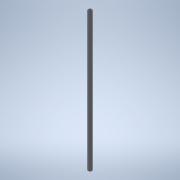
# Autodesk Inventor part: 20-4040_2m
Saved by Autodesk Inventor 2021 (Build 250183000, 183)
## iProperties
Created: 2014-04-23
Part Number: 20-4040_2m
Material: Generic
Document SubType Name: Modeling
Designer: Ross Bowman
Density: 1 g/cm^3
Engineer: Ross Bowman
Catalog Web Link: 8020.net
Vendor: 80/20 Inc.
Appearance: Default
Company: 80/20 Inc.
Material: 6105-T5 Aluminum
Author: Ross Bowman
Keywords: 80/20 , 8020 , T-Slot , Extrusion
Autodesk Inventor part; units mm, degrees
ref_plane "YZ Plane" through (0, 0, 0) normal (1, 0, 0) x (0, 1, 0)
ref_plane "XZ Plane" through (0, 0, 0) normal (0, 1, 0) x (-1, 0, 0)
ref_plane "XY Plane" through (0, 0, 0) normal (0, 0, 1) x (1, 0, 0)
sketch "Sketch1" plane through (0, 0, 0) normal (0, 0, 1) x (1, 0, 0)
  arc A0 (-12.1249, -12.3045) -> (-10.804, -11.9351) centre (-11.5684, -11.748) ccw
  line L0 (-12.3045, -12.1249) -> (-12.1249, -12.3045)
  arc A1 (-11.9351, -10.804) -> (-12.3045, -12.1249) centre (-11.748, -11.5684) ccw
  arc A2 (-11.9351, -9.196) -> (-11.9351, -10.804) centre (-10, -10) ccw
  arc A3 (-12.3045, -7.8751) -> (-11.9351, -9.196) centre (-11.748, -8.4316) ccw
  line L1 (-12.1249, -7.6955) -> (-12.3045, -7.8751)
  arc A4 (-10.804, -8.0649) -> (-12.1249, -7.6955) centre (-11.5684, -8.252) ccw
  arc A5 (-9.196, -8.0649) -> (-10.804, -8.0649) centre (-10, -10) ccw
  arc A6 (-7.8751, -7.6955) -> (-9.196, -8.0649) centre (-8.4316, -8.252) ccw
  line L2 (-7.6955, -7.8751) -> (-7.8751, -7.6955)
  arc A7 (-8.0649, -9.196) -> (-7.6955, -7.8751) centre (-8.252, -8.4316) ccw
  arc A8 (-8.0649, -10.804) -> (-8.0649, -9.196) centre (-10, -10) ccw
  arc A9 (-7.6955, -12.1249) -> (-8.0649, -10.804) centre (-8.252, -11.5684) ccw
  line L3 (-7.8751, -12.3045) -> (-7.6955, -12.1249)
  arc A10 (-9.196, -11.9351) -> (-7.8751, -12.3045) centre (-8.4316, -11.748) ccw
  arc A11 (-10.804, -11.9351) -> (-9.196, -11.9351) centre (-10, -10) ccw
  arc A12 (-2.505, -17.992) -> (-1.997, -18.5) centre (-1.997, -17.992) ccw
  line L4 (-2.505, -16.6448) -> (-2.505, -17.992)
  arc A13 (-2.505, -16.6448) -> (-2.6538, -16.2856) centre (-3.013, -16.6448) ccw
  line L5 (-6.1962, -12.7431) -> (-2.6538, -16.2856)
  arc A14 (-6.345, -12.3839) -> (-6.1962, -12.7431) centre (-5.837, -12.3839) ccw
  line L6 (-6.345, -7.488) -> (-6.345, -12.3839)
  arc A15 (-6.345, -7.488) -> (-7.488, -6.345) centre (-7.488, -7.488) ccw
  line L7 (-12.3839, -6.345) -> (-7.488, -6.345)
  arc A16 (-12.7431, -6.1962) -> (-12.3839, -6.345) centre (-12.3839, -5.837) ccw
  line L8 (-16.2856, -2.6538) -> (-12.7431, -6.1962)
  arc A17 (-16.2856, -2.6538) -> (-16.6448, -2.505) centre (-16.6448, -3.013) ccw
  line L9 (-17.992, -2.505) -> (-16.6448, -2.505)
  arc A18 (-18.5, -1.997) -> (-17.992, -2.505) centre (-17.992, -1.997) ccw
  line L10 (-18.5, 1.997) -> (-18.5, -1.997)
  arc A19 (-17.992, 2.505) -> (-18.5, 1.997) centre (-17.992, 1.997) ccw
  line L11 (-16.6448, 2.505) -> (-17.992, 2.505)
  arc A20 (-16.6448, 2.505) -> (-16.2856, 2.6538) centre (-16.6448, 3.013) ccw
  line L12 (-12.7431, 6.1962) -> (-16.2856, 2.6538)
  arc A21 (-12.3839, 6.345) -> (-12.7431, 6.1962) centre (-12.3839, 5.837) ccw
  line L13 (-7.488, 6.345) -> (-12.3839, 6.345)
  arc A22 (-7.488, 6.345) -> (-6.345, 7.488) centre (-7.488, 7.488) ccw
  line L14 (-6.345, 12.3839) -> (-6.345, 7.488)
  arc A23 (-6.1962, 12.7431) -> (-6.345, 12.3839) centre (-5.837, 12.3839) ccw
  line L15 (-2.6538, 16.2856) -> (-6.1962, 12.7431)
  arc A24 (-2.6538, 16.2856) -> (-2.505, 16.6448) centre (-3.013, 16.6448) ccw
  line L16 (-2.505, 17.992) -> (-2.505, 16.6448)
  arc A25 (-1.997, 18.5) -> (-2.505, 17.992) centre (-1.997, 17.992) ccw
  line L17 (1.997, 18.5) -> (-1.997, 18.5)
  arc A26 (2.505, 17.992) -> (1.997, 18.5) centre (1.997, 17.992) ccw
  line L18 (2.505, 16.6448) -> (2.505, 17.992)
  arc A27 (2.505, 16.6448) -> (2.6538, 16.2856) centre (3.013, 16.6448) ccw
  line L19 (6.1962, 12.7431) -> (2.6538, 16.2856)
  arc A28 (6.345, 12.3839) -> (6.1962, 12.7431) centre (5.837, 12.3839) ccw
  line L20 (6.345, 7.488) -> (6.345, 12.3839)
  arc A29 (6.345, 7.488) -> (7.488, 6.345) centre (7.488, 7.488) ccw
  line L21 (12.3839, 6.345) -> (7.488, 6.345)
  arc A30 (12.7431, 6.1962) -> (12.3839, 6.345) centre (12.3839, 5.837) ccw
  line L22 (16.2856, 2.6538) -> (12.7431, 6.1962)
  arc A31 (16.2856, 2.6538) -> (16.6448, 2.505) centre (16.6448, 3.013) ccw
  line L23 (17.992, 2.505) -> (16.6448, 2.505)
  arc A32 (18.5, 1.997) -> (17.992, 2.505) centre (17.992, 1.997) ccw
  line L24 (18.5, -1.997) -> (18.5, 1.997)
  arc A33 (17.992, -2.505) -> (18.5, -1.997) centre (17.992, -1.997) ccw
  line L25 (16.6448, -2.505) -> (17.992, -2.505)
  arc A34 (16.6448, -2.505) -> (16.2856, -2.6538) centre (16.6448, -3.013) ccw
  line L26 (12.7431, -6.1962) -> (16.2856, -2.6538)
  arc A35 (12.3839, -6.345) -> (12.7431, -6.1962) centre (12.3839, -5.837) ccw
  line L27 (7.488, -6.345) -> (12.3839, -6.345)
  arc A36 (7.488, -6.345) -> (6.345, -7.488) centre (7.488, -7.488) ccw
  line L28 (6.345, -12.3839) -> (6.345, -7.488)
  arc A37 (6.1962, -12.7431) -> (6.345, -12.3839) centre (5.837, -12.3839) ccw
  line L29 (2.6538, -16.2856) -> (6.1962, -12.7431)
  arc A38 (2.6538, -16.2856) -> (2.505, -16.6448) centre (3.013, -16.6448) ccw
  line L30 (2.505, -17.992) -> (2.505, -16.6448)
  arc A39 (1.997, -18.5) -> (2.505, -17.992) centre (1.997, -17.992) ccw
  line L31 (-1.997, -18.5) -> (1.997, -18.5)
  arc A40 (7.8751, -12.3045) -> (9.196, -11.9351) centre (8.4316, -11.748) ccw
  line L32 (7.6955, -12.1249) -> (7.8751, -12.3045)
  arc A41 (8.0649, -10.804) -> (7.6955, -12.1249) centre (8.252, -11.5684) ccw
  arc A42 (8.0649, -9.196) -> (8.0649, -10.804) centre (10, -10) ccw
  arc A43 (7.6955, -7.8751) -> (8.0649, -9.196) centre (8.252, -8.4316) ccw
  line L33 (7.8751, -7.6955) -> (7.6955, -7.8751)
  arc A44 (9.196, -8.0649) -> (7.8751, -7.6955) centre (8.4316, -8.252) ccw
  arc A45 (10.804, -8.0649) -> (9.196, -8.0649) centre (10, -10) ccw
  arc A46 (12.1249, -7.6955) -> (10.804, -8.0649) centre (11.5684, -8.252) ccw
  line L34 (12.3045, -7.8751) -> (12.1249, -7.6955)
  arc A47 (11.9351, -9.196) -> (12.3045, -7.8751) centre (11.748, -8.4316) ccw
  arc A48 (11.9351, -10.804) -> (11.9351, -9.196) centre (10, -10) ccw
  arc A49 (12.3045, -12.1249) -> (11.9351, -10.804) centre (11.748, -11.5684) ccw
  line L35 (12.1249, -12.3045) -> (12.3045, -12.1249)
  arc A50 (10.804, -11.9351) -> (12.1249, -12.3045) centre (11.5684, -11.748) ccw
  arc A51 (9.196, -11.9351) -> (10.804, -11.9351) centre (10, -10) ccw
  arc A52 (-12.1249, 7.6955) -> (-10.804, 8.0649) centre (-11.5684, 8.252) ccw
  line L36 (-12.3045, 7.8751) -> (-12.1249, 7.6955)
  arc A53 (-11.9351, 9.196) -> (-12.3045, 7.8751) centre (-11.748, 8.4316) ccw
  arc A54 (-11.9351, 10.804) -> (-11.9351, 9.196) centre (-10, 10) ccw
  arc A55 (-12.3045, 12.1249) -> (-11.9351, 10.804) centre (-11.748, 11.5684) ccw
  line L37 (-12.1249, 12.3045) -> (-12.3045, 12.1249)
  arc A56 (-10.804, 11.9351) -> (-12.1249, 12.3045) centre (-11.5684, 11.748) ccw
  arc A57 (-9.196, 11.9351) -> (-10.804, 11.9351) centre (-10, 10) ccw
  arc A58 (-7.8751, 12.3045) -> (-9.196, 11.9351) centre (-8.4316, 11.748) ccw
  line L38 (-7.6955, 12.1249) -> (-7.8751, 12.3045)
  arc A59 (-8.0649, 10.804) -> (-7.6955, 12.1249) centre (-8.252, 11.5684) ccw
  arc A60 (-8.0649, 9.196) -> (-8.0649, 10.804) centre (-10, 10) ccw
  arc A61 (-7.6955, 7.8751) -> (-8.0649, 9.196) centre (-8.252, 8.4316) ccw
  line L39 (-7.8751, 7.6955) -> (-7.6955, 7.8751)
  arc A62 (-9.196, 8.0649) -> (-7.8751, 7.6955) centre (-8.4316, 8.252) ccw
  arc A63 (-10.804, 8.0649) -> (-9.196, 8.0649) centre (-10, 10) ccw
  arc A64 (7.8751, 7.6955) -> (9.196, 8.0649) centre (8.4316, 8.252) ccw
  line L40 (7.6955, 7.8751) -> (7.8751, 7.6955)
  arc A65 (8.0649, 9.196) -> (7.6955, 7.8751) centre (8.252, 8.4316) ccw
  arc A66 (8.0649, 10.804) -> (8.0649, 9.196) centre (10, 10) ccw
  arc A67 (7.6955, 12.1249) -> (8.0649, 10.804) centre (8.252, 11.5684) ccw
  line L41 (7.8751, 12.3045) -> (7.6955, 12.1249)
  arc A68 (9.196, 11.9351) -> (7.8751, 12.3045) centre (8.4316, 11.748) ccw
  arc A69 (10.804, 11.9351) -> (9.196, 11.9351) centre (10, 10) ccw
  arc A70 (12.1249, 12.3045) -> (10.804, 11.9351) centre (11.5684, 11.748) ccw
  line L42 (12.3045, 12.1249) -> (12.1249, 12.3045)
  arc A71 (11.9351, 10.804) -> (12.3045, 12.1249) centre (11.748, 11.5684) ccw
  arc A72 (11.9351, 9.196) -> (11.9351, 10.804) centre (10, 10) ccw
  arc A73 (12.3045, 7.8751) -> (11.9351, 9.196) centre (11.748, 8.4316) ccw
  line L43 (12.1249, 7.6955) -> (12.3045, 7.8751)
  arc A74 (10.804, 8.0649) -> (12.1249, 7.6955) centre (11.5684, 8.252) ccw
  arc A75 (9.196, 8.0649) -> (10.804, 8.0649) centre (10, 10) ccw
  arc A76 (-12.3839, -13.655) -> (-12.7431, -13.8038) centre (-12.3839, -14.163) ccw
  line L44 (-12.3839, -13.655) -> (-7.6161, -13.655)
  arc A77 (-7.2569, -13.8038) -> (-7.6161, -13.655) centre (-7.6161, -14.163) ccw
  line L45 (-7.2569, -13.8038) -> (-4.1538, -16.9069)
  arc A78 (-4.005, -17.2661) -> (-4.1538, -16.9069) centre (-4.513, -17.2661) ccw
  line L46 (-4.005, -17.2661) -> (-4.005, -17.992)
  arc A79 (-4.513, -18.5) -> (-4.005, -17.992) centre (-4.513, -17.992) ccw
  line L47 (-4.513, -18.5) -> (-6.862, -18.5)
  arc A80 (-6.862, -18.5) -> (-7.37, -19.008) centre (-6.862, -19.008) ccw
  line L48 (-7.37, -19.008) -> (-7.37, -19.492)
  arc A81 (-7.37, -19.492) -> (-6.862, -20) centre (-6.862, -19.492) ccw
  line L49 (-6.862, -20) -> (6.862, -20)
  arc A82 (6.862, -20) -> (7.37, -19.492) centre (6.862, -19.492) ccw
  line L50 (7.37, -19.492) -> (7.37, -19.008)
  arc A83 (7.37, -19.008) -> (6.862, -18.5) centre (6.862, -19.008) ccw
  line L51 (6.862, -18.5) -> (4.513, -18.5)
  arc A84 (4.005, -17.992) -> (4.513, -18.5) centre (4.513, -17.992) ccw
  line L52 (4.005, -17.992) -> (4.005, -17.2661)
  arc A85 (4.1538, -16.9069) -> (4.005, -17.2661) centre (4.513, -17.2661) ccw
  line L53 (4.1538, -16.9069) -> (7.2569, -13.8038)
  arc A86 (7.6161, -13.655) -> (7.2569, -13.8038) centre (7.6161, -14.163) ccw
  line L54 (7.6161, -13.655) -> (12.3839, -13.655)
  arc A87 (12.7431, -13.8038) -> (12.3839, -13.655) centre (12.3839, -14.163) ccw
  line L55 (12.7431, -13.8038) -> (15.8462, -16.9069)
  arc A88 (15.995, -17.2661) -> (15.8462, -16.9069) centre (15.487, -17.2661) ccw
  line L56 (15.995, -17.2661) -> (15.995, -17.992)
  arc A89 (15.487, -18.5) -> (15.995, -17.992) centre (15.487, -17.992) ccw
  line L57 (15.487, -18.5) -> (13.138, -18.5)
  arc A90 (13.138, -18.5) -> (12.63, -19.008) centre (13.138, -19.008) ccw
  line L58 (12.63, -19.008) -> (12.63, -19.492)
  arc A91 (12.63, -19.492) -> (13.138, -20) centre (13.138, -19.492) ccw
  line L59 (13.138, -20) -> (18.5, -20)
  arc A92 (18.5, -20) -> (20, -18.5) centre (18.5, -18.5) ccw
  line L60 (20, -18.5) -> (20, -13.138)
  arc A93 (20, -13.138) -> (19.492, -12.63) centre (19.492, -13.138) ccw
  line L61 (19.492, -12.63) -> (19.008, -12.63)
  arc A94 (19.008, -12.63) -> (18.5, -13.138) centre (19.008, -13.138) ccw
  line L62 (18.5, -13.138) -> (18.5, -15.487)
  arc A95 (17.992, -15.995) -> (18.5, -15.487) centre (17.992, -15.487) ccw
  line L63 (17.992, -15.995) -> (17.2661, -15.995)
  arc A96 (16.9069, -15.8462) -> (17.2661, -15.995) centre (17.2661, -15.487) ccw
  line L64 (16.9069, -15.8462) -> (13.8038, -12.7431)
  arc A97 (13.655, -12.3839) -> (13.8038, -12.7431) centre (14.163, -12.3839) ccw
  line L65 (13.655, -12.3839) -> (13.655, -7.6161)
  arc A98 (13.8038, -7.2569) -> (13.655, -7.6161) centre (14.163, -7.6161) ccw
  line L66 (13.8038, -7.2569) -> (16.9069, -4.1538)
  arc A99 (17.2661, -4.005) -> (16.9069, -4.1538) centre (17.2661, -4.513) ccw
  line L67 (17.2661, -4.005) -> (17.992, -4.005)
  arc A100 (18.5, -4.513) -> (17.992, -4.005) centre (17.992, -4.513) ccw
  line L68 (18.5, -4.513) -> (18.5, -6.862)
  arc A101 (18.5, -6.862) -> (19.008, -7.37) centre (19.008, -6.862) ccw
  line L69 (19.008, -7.37) -> (19.492, -7.37)
  arc A102 (19.492, -7.37) -> (20, -6.862) centre (19.492, -6.862) ccw
  line L70 (20, -6.862) -> (20, 6.862)
  arc A103 (20, 6.862) -> (19.492, 7.37) centre (19.492, 6.862) ccw
  line L71 (19.492, 7.37) -> (19.008, 7.37)
  arc A104 (19.008, 7.37) -> (18.5, 6.862) centre (19.008, 6.862) ccw
  line L72 (18.5, 6.862) -> (18.5, 4.513)
  arc A105 (17.992, 4.005) -> (18.5, 4.513) centre (17.992, 4.513) ccw
  line L73 (17.992, 4.005) -> (17.2661, 4.005)
  arc A106 (16.9069, 4.1538) -> (17.2661, 4.005) centre (17.2661, 4.513) ccw
  line L74 (16.9069, 4.1538) -> (13.8038, 7.2569)
  arc A107 (13.655, 7.6161) -> (13.8038, 7.2569) centre (14.163, 7.6161) ccw
  line L75 (13.655, 7.6161) -> (13.655, 12.3839)
  arc A108 (13.8038, 12.7431) -> (13.655, 12.3839) centre (14.163, 12.3839) ccw
  line L76 (13.8038, 12.7431) -> (16.9069, 15.8462)
  arc A109 (17.2661, 15.995) -> (16.9069, 15.8462) centre (17.2661, 15.487) ccw
  line L77 (17.2661, 15.995) -> (17.992, 15.995)
  arc A110 (18.5, 15.487) -> (17.992, 15.995) centre (17.992, 15.487) ccw
  line L78 (18.5, 15.487) -> (18.5, 13.138)
  arc A111 (18.5, 13.138) -> (19.008, 12.63) centre (19.008, 13.138) ccw
  line L79 (19.008, 12.63) -> (19.492, 12.63)
  arc A112 (19.492, 12.63) -> (20, 13.138) centre (19.492, 13.138) ccw
  line L80 (20, 13.138) -> (20, 18.5)
  arc A113 (20, 18.5) -> (18.5, 20) centre (18.5, 18.5) ccw
  line L81 (18.5, 20) -> (13.138, 20)
  arc A114 (13.138, 20) -> (12.63, 19.492) centre (13.138, 19.492) ccw
  line L82 (12.63, 19.492) -> (12.63, 19.008)
  arc A115 (12.63, 19.008) -> (13.138, 18.5) centre (13.138, 19.008) ccw
  line L83 (13.138, 18.5) -> (15.487, 18.5)
  arc A116 (15.995, 17.992) -> (15.487, 18.5) centre (15.487, 17.992) ccw
  line L84 (15.995, 17.992) -> (15.995, 17.2661)
  arc A117 (15.8462, 16.9069) -> (15.995, 17.2661) centre (15.487, 17.2661) ccw
  line L85 (15.8462, 16.9069) -> (12.7431, 13.8038)
  arc A118 (12.3839, 13.655) -> (12.7431, 13.8038) centre (12.3839, 14.163) ccw
  line L86 (12.3839, 13.655) -> (7.6161, 13.655)
  arc A119 (7.2569, 13.8038) -> (7.6161, 13.655) centre (7.6161, 14.163) ccw
  line L87 (7.2569, 13.8038) -> (4.1538, 16.9069)
  arc A120 (4.005, 17.2661) -> (4.1538, 16.9069) centre (4.513, 17.2661) ccw
  line L88 (4.005, 17.2661) -> (4.005, 17.992)
  arc A121 (4.513, 18.5) -> (4.005, 17.992) centre (4.513, 17.992) ccw
  line L89 (4.513, 18.5) -> (6.862, 18.5)
  arc A122 (6.862, 18.5) -> (7.37, 19.008) centre (6.862, 19.008) ccw
  line L90 (7.37, 19.008) -> (7.37, 19.492)
  arc A123 (7.37, 19.492) -> (6.862, 20) centre (6.862, 19.492) ccw
  line L91 (6.862, 20) -> (-6.862, 20)
  arc A124 (-6.862, 20) -> (-7.37, 19.492) centre (-6.862, 19.492) ccw
  line L92 (-7.37, 19.492) -> (-7.37, 19.008)
  arc A125 (-7.37, 19.008) -> (-6.862, 18.5) centre (-6.862, 19.008) ccw
  line L93 (-6.862, 18.5) -> (-4.513, 18.5)
  arc A126 (-4.005, 17.992) -> (-4.513, 18.5) centre (-4.513, 17.992) ccw
  line L94 (-4.005, 17.992) -> (-4.005, 17.2661)
  arc A127 (-4.1538, 16.9069) -> (-4.005, 17.2661) centre (-4.513, 17.2661) ccw
  line L95 (-4.1538, 16.9069) -> (-7.2569, 13.8038)
  arc A128 (-7.6161, 13.655) -> (-7.2569, 13.8038) centre (-7.6161, 14.163) ccw
  line L96 (-7.6161, 13.655) -> (-12.3839, 13.655)
  arc A129 (-12.7431, 13.8038) -> (-12.3839, 13.655) centre (-12.3839, 14.163) ccw
  line L97 (-12.7431, 13.8038) -> (-15.8462, 16.9069)
  arc A130 (-15.995, 17.2661) -> (-15.8462, 16.9069) centre (-15.487, 17.2661) ccw
  line L98 (-15.995, 17.2661) -> (-15.995, 17.992)
  arc A131 (-15.487, 18.5) -> (-15.995, 17.992) centre (-15.487, 17.992) ccw
  line L99 (-15.487, 18.5) -> (-13.138, 18.5)
  arc A132 (-13.138, 18.5) -> (-12.63, 19.008) centre (-13.138, 19.008) ccw
  line L100 (-12.63, 19.008) -> (-12.63, 19.492)
  arc A133 (-12.63, 19.492) -> (-13.138, 20) centre (-13.138, 19.492) ccw
  line L101 (-13.138, 20) -> (-18.5, 20)
  arc A134 (-18.5, 20) -> (-20, 18.5) centre (-18.5, 18.5) ccw
  line L102 (-20, 18.5) -> (-20, 13.138)
  arc A135 (-20, 13.138) -> (-19.492, 12.63) centre (-19.492, 13.138) ccw
  line L103 (-19.492, 12.63) -> (-19.008, 12.63)
  arc A136 (-19.008, 12.63) -> (-18.5, 13.138) centre (-19.008, 13.138) ccw
  line L104 (-18.5, 13.138) -> (-18.5, 15.487)
  arc A137 (-17.992, 15.995) -> (-18.5, 15.487) centre (-17.992, 15.487) ccw
  line L105 (-17.992, 15.995) -> (-17.2661, 15.995)
  arc A138 (-16.9069, 15.8462) -> (-17.2661, 15.995) centre (-17.2661, 15.487) ccw
  line L106 (-16.9069, 15.8462) -> (-13.8038, 12.7431)
  arc A139 (-13.655, 12.3839) -> (-13.8038, 12.7431) centre (-14.163, 12.3839) ccw
  line L107 (-13.655, 12.3839) -> (-13.655, 7.6161)
  arc A140 (-13.8038, 7.2569) -> (-13.655, 7.6161) centre (-14.163, 7.6161) ccw
  line L108 (-13.8038, 7.2569) -> (-16.9069, 4.1538)
  arc A141 (-17.2661, 4.005) -> (-16.9069, 4.1538) centre (-17.2661, 4.513) ccw
  line L109 (-17.2661, 4.005) -> (-17.992, 4.005)
  arc A142 (-18.5, 4.513) -> (-17.992, 4.005) centre (-17.992, 4.513) ccw
  line L110 (-18.5, 4.513) -> (-18.5, 6.862)
  arc A143 (-18.5, 6.862) -> (-19.008, 7.37) centre (-19.008, 6.862) ccw
  line L111 (-19.008, 7.37) -> (-19.492, 7.37)
  arc A144 (-19.492, 7.37) -> (-20, 6.862) centre (-19.492, 6.862) ccw
  line L112 (-20, 6.862) -> (-20, -6.862)
  arc A145 (-20, -6.862) -> (-19.492, -7.37) centre (-19.492, -6.862) ccw
  line L113 (-19.492, -7.37) -> (-19.008, -7.37)
  arc A146 (-19.008, -7.37) -> (-18.5, -6.862) centre (-19.008, -6.862) ccw
  line L114 (-18.5, -6.862) -> (-18.5, -4.513)
  arc A147 (-17.992, -4.005) -> (-18.5, -4.513) centre (-17.992, -4.513) ccw
  line L115 (-17.992, -4.005) -> (-17.2661, -4.005)
  arc A148 (-16.9069, -4.1538) -> (-17.2661, -4.005) centre (-17.2661, -4.513) ccw
  line L116 (-16.9069, -4.1538) -> (-13.8038, -7.2569)
  arc A149 (-13.655, -7.6161) -> (-13.8038, -7.2569) centre (-14.163, -7.6161) ccw
  line L117 (-13.655, -7.6161) -> (-13.655, -12.3839)
  arc A150 (-13.8038, -12.7431) -> (-13.655, -12.3839) centre (-14.163, -12.3839) ccw
  line L118 (-13.8038, -12.7431) -> (-16.9069, -15.8462)
  arc A151 (-17.2661, -15.995) -> (-16.9069, -15.8462) centre (-17.2661, -15.487) ccw
  line L119 (-17.2661, -15.995) -> (-17.992, -15.995)
  arc A152 (-18.5, -15.487) -> (-17.992, -15.995) centre (-17.992, -15.487) ccw
  line L120 (-18.5, -15.487) -> (-18.5, -13.138)
  arc A153 (-18.5, -13.138) -> (-19.008, -12.63) centre (-19.008, -13.138) ccw
  line L121 (-19.008, -12.63) -> (-19.492, -12.63)
  arc A154 (-19.492, -12.63) -> (-20, -13.138) centre (-19.492, -13.138) ccw
  line L122 (-20, -13.138) -> (-20, -18.5)
  arc A155 (-20, -18.5) -> (-18.5, -20) centre (-18.5, -18.5) ccw
  line L123 (-18.5, -20) -> (-13.138, -20)
  arc A156 (-13.138, -20) -> (-12.63, -19.492) centre (-13.138, -19.492) ccw
  line L124 (-12.63, -19.492) -> (-12.63, -19.008)
  arc A157 (-12.63, -19.008) -> (-13.138, -18.5) centre (-13.138, -19.008) ccw
  line L125 (-13.138, -18.5) -> (-15.487, -18.5)
  arc A158 (-15.995, -17.992) -> (-15.487, -18.5) centre (-15.487, -17.992) ccw
  line L126 (-15.995, -17.992) -> (-15.995, -17.2661)
  arc A159 (-15.8462, -16.9069) -> (-15.995, -17.2661) centre (-15.487, -17.2661) ccw
  line L127 (-15.8462, -16.9069) -> (-12.7431, -13.8038)
  point P0 (0, 0)
  constraints: 320 point on circle, 256 end point, 160 centre point
extrude "Extrusion1" add sketch "Sketch1" against normal blind 100
move faces "Move1" translate (0, 0, 1900) faces at (-0.6657, 19.5, 0)
body "Solid1"
